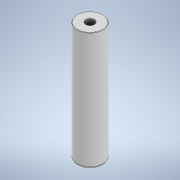
# Autodesk Inventor part: 74. Ось блока заднего хода
Saved by Autodesk Inventor 2021 (Build 250183000, 183)
## iProperties
Created: 2021-03-11
Part Number: 74. Ось блока заднего хода
Material: Типовые
Document SubType Name: Modeling
Designer: Данил
Density: 1 g/cm^3
Appearance: По умолчанию
Author: Данил
Autodesk Inventor part; units mm, degrees
ref_plane "YZ Plane" through (0, 0, 0) normal (1, 0, 0) x (0, 1, 0)
ref_plane "XZ Plane" through (0, 0, 0) normal (0, 1, 0) x (-1, 0, 0)
ref_plane "XY Plane" through (0, 0, 0) normal (0, 0, 1) x (1, 0, 0)
sketch "Эскиз1" plane through (0, 0, 0) normal (0, 0, 1) x (1, 0, 0)
  line L0 (0, 57) -> (0, -57)
  line L1 (0, -57) -> (11.634, -57)
  line L2 (11.634, -57) -> (12.5, -55.5)
  line L3 (12.5, -55.5) -> (12.5, 43)
  line L4 (12.5, 43) -> (12.5, 43)
  line L5 (12.5, 43) -> (12.5, 56.5)
  line L6 (12.2113, 57) -> (0, 57)
  line L7 (12.5, 56.5) -> (12.2113, 57)
  point P0 (0, 0)
  point P1 (0, 0)
  point P2 (12.5, 57)
  point P3 (12.5, 43)
  dimension "d0" = 114
  dimension "d1" = 30
  dimension "d2" = 25
  dimension "d3" = 1.5
  dimension "d4" = 100
  dimension "d5" = 25
  dimension "d6" = 0.5
  dimension "d7" = 30
  constraints: 16 end point, 3 horizontal, 2 perpendicular, 2 point on line, 1 coincident, 1 midpoint, 1 vertical
  measures "d0" distance of L0.start L0.end
  measures "d1" angle of L3 L2
  measures "d2" diameter of L3 L0
  measures "d3" distance from line of L2.end L1
  measures "d4" distance from line of L1 L3.end
  measures "d5" diameter of L5 L0
  measures "d6" distance of L5.end point (12.5, 57)
  measures "d7" angle of L5 L7
revolve "Вращение1" add sketch "Эскиз1" angle 360 about axis through (0, 57, 0) along (0, -1, 0)
sketch "Эскиз3" plane through (0, 57, 0) normal (0, 1, 0) x (1, 0, 0)
  circle A0 centre (0, 0) radius 12.2113 projected
  point P0 (0, 0)
  constraints: 1 coincident
hole "Отверстие1" at (0, 57, 0) direction (0, -1, 0) diameter 8.376 depth 25 tip angle 120 countersink diameter 8.4 countersink angle 90 thread size "M10x1.5" class "6H" standard "ISO Metric profile"
